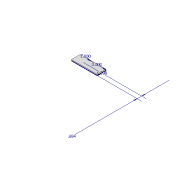
# Autodesk Inventor part: capstone hook mount
Saved by Autodesk Inventor 2020 (Build 240168000, 168)
## iProperties
Created: 2020-02-12
Part Number: capstone hook mount
Material: Generic
Document SubType Name: Modeling
Designer: ball
Density: 1 g/cm^3
Appearance: Default
Author: ball
Autodesk Inventor part; units mm, degrees
ref_plane "YZ Plane" through (0, 0, 0) normal (1, 0, 0) x (0, 1, 0)
ref_plane "XZ Plane" through (0, 0, 0) normal (0, 1, 0) x (-1, 0, 0)
ref_plane "XY Plane" through (0, 0, 0) normal (0, 0, 1) x (1, 0, 0)
sketch "Sketch1" plane through (0, 0, 0) normal (0, 1, 0) x (-1, 0, 0)
  line L0 (0, 17.637) -> (-76.2, 17.637)
  line L1 (-76.2, 17.637) -> (-76.2, -17.863)
  line L2 (-76.2, -17.863) -> (0, -17.863)
  line L3 (0, -17.863) -> (0, 17.637)
  line L4 (0, 17.637) -> (25.4, 17.637)
  line L5 (25.4, 17.637) -> (25.4, -17.863)
  line L6 (25.4, -17.863) -> (0, -17.863)
  line L7 (0, -17.863) -> (0, 17.637)
  point P0 (0, 0)
  dimension "d0" = 76.2
  dimension "d1" = 35.5
  dimension "d2" = 17.637
  dimension "d3" = 25.4
  constraints: 16 end point, 4 parallel, 2 horizontal, 2 perpendicular
  measures "d0" distance of L2.end L1.end
  measures "d1" distance of L1.end L0.end
  measures "d2" distance from line of L0 point (0, 0)
  measures "d3" distance of L5.end L6.end
extrude "Extrusion1" add sketch "Sketch1" along normal blind 4
body "Solid1"
